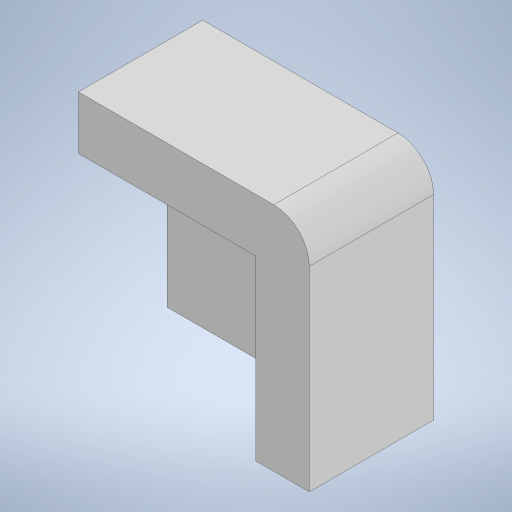
# Autodesk Inventor part: pièce_intérieur_coque_RPI
Saved by Autodesk Inventor 2023 (Build 270158000, 158)
## iProperties
Created: 2023-03-28
Part Number: pièce_intérieur_coque_RPI
Material: Générique
Document SubType Name: Modeling
Designer: egozi
Density: 1 g/cm^3
Appearance: Par défaut
Author: egozi
Autodesk Inventor part; units mm, degrees
ref_plane "YZ Plane" through (0, 0, 0) normal (1, 0, 0) x (0, 1, 0)
ref_plane "XZ Plane" through (0, 0, 0) normal (0, 1, 0) x (-1, 0, 0)
ref_plane "XY Plane" through (0, 0, 0) normal (0, 0, 1) x (1, 0, 0)
sketch "Esquisse1" plane through (0, 0, 0) normal (0, 0, 1) x (1, 0, 0)
  line L0 (0, -2.6) -> (0, 15.6) projected
  line L1 (-12.6, 0) -> (5.6, 0) projected
  line L2 (-10, 10) -> (0, 10)
  line L3 (0, 10) -> (0, 0)
  line L4 (0, 0) -> (-10, 0)
  line L5 (-10, 0) -> (-10, 10)
  line L6 (-10, 10) -> (0, 10)
  line L7 (0, 10) -> (0, 13)
  line L8 (0, 13) -> (-10, 13)
  line L9 (-10, 13) -> (-10, 10)
  line L10 (0, 0) -> (3, 0)
  line L11 (3, 0) -> (3, 13)
  line L12 (3, 13) -> (0, 13)
  line L13 (0, 13) -> (0, 0)
  dimension "d0" = 10
  dimension "d1" = 10
  dimension "d2" = 3
  dimension "d3" = 3
  constraints: 24 end point, 6 parallel, 3 horizontal, 3 perpendicular, 3 point on line, 1 collinear
  measures "d0" distance of L2.start L2.end
  measures "d1" distance of L4.end L2.start
  measures "d2" distance of L8.end L2.start
  measures "d3" distance of L11.end L12.end
extrude "Extrusion1" add sketch "Esquisse1" along normal blind 2
sketch "Esquisse2" plane through (0, 0, 2) normal (0, 0, 1) x (1, 0, 0)
  line L0 (3, 13) -> (-10, 13) projected
  line L1 (3, 0) -> (3, 13) projected
  line L2 (-10, 13) -> (3, 13)
  line L3 (3, 13) -> (3, 10)
  line L4 (3, 10) -> (-10, 10)
  line L5 (-10, 10) -> (-10, 13)
  line L6 (3, 0) -> (0, 0)
  line L7 (0, 0) -> (0, 10)
  line L8 (0, 10) -> (3, 10)
  line L9 (3, 10) -> (3, 0)
  dimension "d6" = 3
  dimension "d7" = 3
  constraints: 16 end point, 4 parallel, 2 horizontal, 2 perpendicular, 2 point on line
  measures "d6" distance of L4.end L0.end
  measures "d7" distance of L1.start L6.end
extrude "Extrusion2" add sketch "Esquisse2" along normal blind 5
fillet "Congé1" radius 2 1 edges at (3, 13, 3.5)
